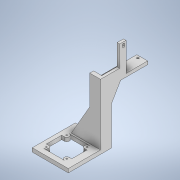
# Autodesk Inventor part: camera_mount_v1
Saved by Autodesk Inventor 2022 (Build 260153000, 153)
## iProperties
Created: 2022-06-05
Part Number: camera_mount_v1
Material: Generic
Document SubType Name: Modeling
Designer: kylem
Density: 1 g/cm^3
Appearance: Default
Author: kylem
Autodesk Inventor part; units mm, degrees
ref_plane "YZ Plane" through (0, 0, 0) normal (1, 0, 0) x (0, 1, 0)
ref_plane "XZ Plane" through (0, 0, 0) normal (0, 1, 0) x (-1, 0, 0)
ref_plane "XY Plane" through (0, 0, 0) normal (0, 0, 1) x (1, 0, 0)
sketch "Sketch1" plane through (0, 0, 0) normal (0, 1, 0) x (-1, 0, 0)
  line L0 (0, 0) -> (13, 0)
  line L1 (13, 0) -> (13, -44)
  line L2 (13, -44) -> (0, -44)
  line L3 (0, -44) -> (0, 0)
  line L4 (13, 0) -> (13, -6)
  line L5 (13, -6) -> (7.5, -6)
  line L6 (7.5, -6) -> (7.5, -40)
  circle A0 centre (7.5, -6) radius 1.6
  circle A1 centre (7.5, -40) radius 1.6
  dimension "d0" = 13
  dimension "d1" = 44
  dimension "d2" = 6
  dimension "d3" = 5.5
  dimension "d4" = 34
  dimension "d5" = 3.2
  dimension "d6" = 3.2
  constraints: 14 end point, 3 parallel, 2 centre point, 2 coincident, 2 perpendicular, 1 horizontal, 1 point on line
  measures "d0" distance of L1.end L2.end
  measures "d1" distance of L0.end L1.end
  measures "d2" distance of L0.end L4.end
  measures "d3" distance of L4.end L5.end
  measures "d4" distance of L5.end L6.end
  measures "d5" diameter of A0
  measures "d6" diameter of A1
extrude "Extrusion1" add sketch "Sketch1" along normal blind 5
sketch "Sketch2" plane through (0, 0, 0) normal (1, 0, 0) x (0, 0, -1)
  line L0 (0, 5) -> (44, 5) projected
  line L1 (0, 5) -> (44, 5)
  line L2 (44, 5) -> (44, 50)
  line L3 (44, 50) -> (0, 50)
  line L4 (0, 50) -> (0, 5)
  line L5 (0, 0) -> (44, 0)
  line L6 (44, 0) -> (44, 5)
  line L7 (44, 5) -> (0, 5)
  line L8 (0, 5) -> (0, 0)
  line L9 (0, 50) -> (10, 50)
  line L10 (10, 50) -> (10, 5)
  line L11 (10, 5) -> (0, 5)
  line L12 (0, 5) -> (0, 50)
  dimension "d9" = 44
  dimension "d10" = 45
  dimension "d11" = 10
  constraints: 24 end point, 6 parallel, 3 horizontal, 3 perpendicular, 1 point on line
  measures "d9" distance of L3.end L2.end
  measures "d10" distance of L2.end L1.end
  measures "d11" distance of L10.end L11.end
extrude "Extrusion2" add sketch "Sketch2" along normal blind 4 contours L4 L3 L10 L0 | L0 L6 L5 L8
sketch "Sketch3" plane through (4, 0, 0) normal (1, 0, 0) x (0, 0, -1)
  line L0 (44, 5) -> (10, 5) projected
  line L1 (10, 5) -> (10, 45)
  line L2 (10, 5) -> (10, 50) projected
  line L3 (0, 50) -> (0, 5) projected
  line L4 (0, 45) -> (4.4, 45)
  line L5 (6, 45) -> (6, 46.5)
  line L6 (6, 45) -> (6, 43.5)
  line L7 (4.4, 46.5) -> (4.4, 43.5)
  line L8 (7.6, 46.5) -> (7.6, 43.5)
  arc A0 (5.4432, 45) -> (6, 44.9) centre (6, 46.5) ccw
  arc A1 (6.5568, 45) -> (4.4, 46.5) centre (6, 46.5) ccw
  line L9 (10, 45) -> (6.5568, 45)
  line L10 (5.4432, 45) -> (0, 45)
  arc A2 (6, 45.1) -> (5.4432, 45) centre (6, 43.5) ccw
  arc A3 (4.4, 43.5) -> (7.6, 43.5) centre (6, 43.5) ccw
  point P0 (0, 0)
  dimension "d14" = 40
  dimension "d15" = 6
  dimension "d16" = 1.5
  dimension "d17" = 1.5
  constraints: 16 end point, 9 point on circle, 4 centre point, 4 tangent, 3 point on line, 2 coincident, 2 perpendicular, 2 vertical, 1 midpoint
  measures "d14" distance of L0.end L1.end
  measures "d15" distance of L4.start L5.start
  measures "d16" distance of L5.start L5.end
  measures "d17" distance of L5.start L6.end
extrude "Extrusion3" cut sketch "Sketch3" against normal blind 4 contours L6 A0 A2 L5 | A1 L9 L8 A3 L7 | L8 L9 A1
sketch "Sketch4" plane through (-13, 0, 0) normal (0, 0, 1) x (1, 0, 0)
  line L0 (0, 0) -> (17, 0) projected
  line L1 (17, 0) -> (17, 5) projected
  line L2 (0, 0) -> (17, 0)
  line L3 (17, 0) -> (17, 5)
  line L4 (17, 5) -> (0, 5)
  line L5 (0, 5) -> (0, 0)
  line L6 (13, 50) -> (13, 5) projected
  line L7 (17, 0) -> (13, 0)
  line L8 (13, 0) -> (13, 17)
  line L9 (13, 17) -> (17, 17)
  line L10 (17, 17) -> (17, 0)
  dimension "d22" = 17
  constraints: 16 end point, 4 parallel, 2 horizontal, 2 perpendicular, 1 point on line
  measures "d22" distance of L7.end L8.end
extrude "Extrusion4" add sketch "Sketch4" along normal blind 30
sketch "Sketch5" plane through (0, 0, 0) normal (0, -1, 0) x (1, 0, 0)
  line L0 (-13, -44) -> (-13, 30) projected
  line L1 (-13, 30) -> (4, 30)
  line L2 (4, 30) -> (4, 13)
  line L3 (4, 13) -> (-13, 13)
  line L4 (-13, 13) -> (-13, 30)
  point P0 (0, 0)
  dimension "d25" = 17
  dimension "d26" = 17
  constraints: 8 end point, 2 parallel, 1 horizontal, 1 perpendicular
  measures "d25" distance of L2.end L3.end
  measures "d26" distance of L1.end L2.end
extrude "Extrusion5" add sketch "Sketch5" along normal blind 85
sketch "Sketch7" plane through (0, -85, 0) normal (0, -1, 0) x (1, 0, 0)
  line L0 (4, 13) -> (-13, 13) projected
  line L1 (0, 30) -> (0, -10) projected
  line L2 (0, 13) -> (0, 30)
  line L3 (0, 30) -> (0, 52.6)
  circle A0 centre (-36, 52.6) radius 9
  line L4 (-36, 52.6) -> (-36, 36.6)
  line L5 (-36, 36.6) -> (-20, 36.6)
  line L6 (-36, 52.6) -> (-36, 68.6)
  line L7 (-36, 68.6) -> (-52, 68.6)
  line L8 (-52, 68.6) -> (-20, 68.6)
  line L9 (-20, 68.6) -> (-20, 36.6)
  line L10 (-20, 36.6) -> (-52, 36.6)
  line L11 (-52, 36.6) -> (-52, 68.6)
  circle A1 centre (-20, 68.6) radius 1.1
  circle A2 centre (-20, 36.6) radius 1.1
  circle A3 centre (-52, 36.6) radius 1.1
  circle A4 centre (-52, 68.6) radius 1.1
  circle A5 centre (-20, 68.6) radius 4
  circle A6 centre (-20, 36.6) radius 4
  line L12 (-52, 65.6) -> (-52, 70.6)
  line L13 (-52, 36.6) -> (-52, 42.6)
  circle A7 centre (-52, 68.6) radius 4
  circle A8 centre (-52, 36.6) radius 4
  point P0 (0, 0)
  point P1 (-20, 64.6)
  point P2 (-20, 40.6)
  dimension "d29" = 22.6
  dimension "d31" = 18
  dimension "d32" = 16
  dimension "d33" = 16
  dimension "d34" = 16
  dimension "d35" = 16
  dimension "d36" = 2.2
  dimension "d37" = 2.2
  dimension "d39" = 2.2
  dimension "d40" = 8
  dimension "d43" = 8
  dimension "d49" = 8
  dimension "d50" = 8
  constraints: 24 end point, 9 centre point, 8 coincident, 3 perpendicular, 3 point on line, 2 parallel, 2 vertical, 1 collinear, 1 horizontal
  measures "d29" distance of L1.start L3.end
  measures "d31" diameter of A0
  measures "d32" distance of L4.start L4.end
  measures "d33" distance of L4.end L5.end
  measures "d34" distance of L4.start L6.end
  measures "d35" distance of L6.end L7.end
  measures "d36" diameter of A1
  measures "d37" diameter of A2
  measures "d39" diameter of A4
  measures "d40" diameter of A5
  measures "d43" diameter of A6
  measures "d49" diameter of A7
  measures "d50" diameter of A8
sketch "Sketch14" plane through (0, -85, 0) normal (0, -1, 0) x (1, 0, 0)
  line L0 (4, 13) -> (4, 30) projected
  line L1 (4, 13) -> (4, 52.6)
  line L2 (4, 52.6) -> (-26.5, 52.6)
  line L3 (-26.5, 52.6) -> (-26.5, 36.6)
  line L4 (-26.5, 36.6) -> (-10.5, 36.6)
  line L5 (-26.5, 52.6) -> (-42.5, 52.6)
  line L6 (-42.5, 52.6) -> (-42.5, 68.6)
  line L7 (-42.5, 68.6) -> (-10.5, 68.6)
  line L8 (-10.5, 68.6) -> (-10.5, 36.6)
  line L9 (-10.5, 36.6) -> (-42.5, 36.6)
  line L10 (-42.5, 36.6) -> (-42.5, 68.6)
  circle A0 centre (-42.5, 68.6) radius 1.1
  circle A1 centre (-10.5, 68.6) radius 1.1
  circle A2 centre (-10.5, 36.6) radius 1.1
  circle A3 centre (-42.5, 36.6) radius 1.1
  circle A4 centre (-42.5, 68.6) radius 4
  circle A5 centre (-10.5, 68.6) radius 4
  circle A6 centre (-10.5, 36.6) radius 4
  circle A7 centre (-42.5, 36.6) radius 4
  point P0 (0, 0)
  dimension "d91" = 39.6
  dimension "d92" = 30.5
  dimension "d93" = 16
  dimension "d94" = 16
  dimension "d95" = 16
  dimension "d96" = 16
  dimension "d97" = 2.2
  dimension "d98" = 2.2
  dimension "d99" = 2.2
  dimension "d100" = 2.2
  dimension "d101" = 8
  dimension "d102" = 8
  dimension "d103" = 8
  dimension "d104" = 8
  constraints: 20 end point, 8 centre point, 8 coincident, 4 perpendicular, 2 horizontal, 2 parallel, 1 collinear, 1 vertical
  measures "d91" distance of L0.start L1.end
  measures "d92" distance of L1.end L2.end
  measures "d93" distance of L2.end L3.end
  measures "d94" distance of L3.end L4.end
  measures "d95" distance of L2.end L5.end
  measures "d96" distance of L5.end L6.end
  measures "d97" diameter of A0
  measures "d98" diameter of A1
  measures "d99" diameter of A2
  measures "d100" diameter of A3
  measures "d101" diameter of A4
  measures "d102" diameter of A5
  measures "d103" diameter of A6
  measures "d104" diameter of A7
extrude "Extrusion14" add sketch "Sketch14" against normal blind 6 contours A5 L7 A1 L8 | L8 A1 L7 A5 | A6 L4 A2 L8 | L8 A2 L4 A6 | A7 L10 A3 L9 | L9 A3 L10 A7 | A4 L7 A0 L6 | L6 A0 L7 A4
sketch "Sketch15" plane through (-10.5, -85, 68.6) normal (0, -1, 0) x (1, 0, 0)
  circle A0 centre (0, 0) radius 4 projected
  line L0 (0, 4) -> (10, 4)
  line L1 (10, 4) -> (10, -4)
  line L2 (10, -4) -> (0, -4)
  line L3 (0, -4) -> (0, 4)
  circle A1 centre (0, -32) radius 4 projected
  line L4 (0, -28) -> (10, -28)
  line L5 (10, -28) -> (10, -36)
  line L6 (10, -36) -> (0, -36)
  line L7 (0, -36) -> (0, -28)
  circle A2 centre (-32, -32) radius 4 projected
  line L8 (-32, -36) -> (-42, -36)
  line L9 (-42, -36) -> (-42, -28)
  line L10 (-42, -28) -> (-32, -28)
  line L11 (-32, -28) -> (-32, -36)
  circle A3 centre (-32, 0) radius 4 projected
  line L12 (-32, -4) -> (-42, -4)
  line L13 (-42, -4) -> (-42, 4)
  line L14 (-42, 4) -> (-32, 4)
  line L15 (-32, 4) -> (-32, -4)
  line L16 (-42, 4) -> (-36, 4)
  line L17 (-36, 4) -> (-36, -36)
  line L18 (-36, -36) -> (-42, -36)
  line L19 (-42, -36) -> (-42, 4)
  line L20 (10, 4) -> (4, 4)
  line L21 (4, 4) -> (4, -36)
  line L22 (4, -36) -> (10, -36)
  line L23 (10, -36) -> (10, 4)
  point P0 (10.5, -68.6)
  point P1 (-36, -4)
  point P2 (-32, 4)
  point P3 (-42, -4)
  point P4 (-36, -28)
  point P5 (0, -4)
  point P6 (4, -4)
  point P7 (4, -28)
  point P8 (10, -4)
  dimension "d107" = 10
  dimension "d108" = 8
  dimension "d109" = 10
  dimension "d110" = 8
  dimension "d111" = 10
  dimension "d112" = 8
  dimension "d113" = 10
  dimension "d114" = 8
  dimension "d115" = 6
  dimension "d116" = 6
  constraints: 48 end point, 12 parallel, 6 horizontal, 6 perpendicular, 5 point on line, 8 other
  measures "d107" distance of L1.end L2.end
  measures "d108" distance of L0.end L1.end
  measures "d109" distance of L5.end L6.end
  measures "d110" distance of L4.end L5.end
  measures "d111" distance of L9.end L10.end
  measures "d112" distance of L8.end L9.end
  measures "d113" distance of L13.end L14.end
  measures "d114" distance of L12.end L13.end
  measures "d115" distance of L17.end L18.end
  measures "d116" distance of L22.end L21.end
extrude "Extrusion15" add sketch "Sketch15" against normal blind 6 contours L21 L2 A0 | A0 L0 L21 | L21 L0 L1 L2 | L2 L23 L4 L21 | L21 A1 L4 | L4 L5 L6 L21 | L21 L6 A1 | A2 L17 L10 | L8 L17 A2 | L17 L8 L9 L10 | L10 L19 L12 L17 | L17 A3 L12 | L12 L13 L14 L17 | L17 L14 A3
sketch "Sketch16" plane through (0, -85, 0) normal (0, -1, 0) x (1, 0, 0)
  line L0 (-0.5, 72.6) -> (-0.5, 32.6) projected
  line L1 (-0.5, 72.6) -> (-52.5, 72.6)
  line L2 (-52.5, 72.6) -> (-52.5, 80.6)
  line L3 (-52.5, 80.6) -> (-0.5, 80.6)
  line L4 (-0.5, 80.6) -> (-0.5, 72.6)
  line L5 (-0.5, 32.6) -> (-10.5, 32.6) projected
  line L6 (-0.5, 32.6) -> (-52.5, 32.6)
  line L7 (-52.5, 32.6) -> (-52.5, 24.6)
  line L8 (-52.5, 24.6) -> (-0.5, 24.6)
  line L9 (-0.5, 24.6) -> (-0.5, 32.6)
  point P0 (0, 0)
  dimension "d119" = 8
  dimension "d120" = 8
  constraints: 16 end point, 4 parallel, 2 horizontal, 2 perpendicular
  measures "d119" distance of L1.end L2.end
  measures "d120" distance of L7.end L6.end
extrude "Extrusion16" add sketch "Sketch16" against normal blind 6
sketch "Sketch17" plane through (0, -79, 0) normal (0, 1, 0) x (1, 0, 0)
  line L0 (-0.5, -80.6) -> (-0.5, -30) projected
  line L1 (4, -30) -> (0, -30) projected
  line L2 (-0.5, -80.6) -> (4, -80.6)
  line L3 (4, -80.6) -> (4, -30)
  line L4 (4, -30) -> (-0.5, -30)
  line L5 (-0.5, -30) -> (-0.5, -80.6)
  line L6 (-52.5, -24.6) -> (-52.5, -80.6) projected
  line L7 (-52.5, -24.6) -> (-13, -24.6)
  line L8 (-13, -24.6) -> (-13, -13)
  line L9 (-13, -13) -> (-52.5, -13)
  line L10 (-52.5, -13) -> (-52.5, -24.6)
  point P0 (0, 0)
  constraints: 16 end point, 4 parallel, 2 horizontal, 2 perpendicular
extrude "Extrusion17" add sketch "Sketch17" against normal blind 6
chamfer "Chamfer4" distance 50 angle 30 1 edges at (-13, -79, 21.5) measured on face at (-13, -24.6667, 24.3333)
chamfer "Chamfer5" distance 25 angle 30 1 edges at (-4.5, 0, 13) measured on face at (-16.9558, -64.3333, 13)
sketch "Sketch19" plane through (-13, 0, 30) normal (0, 0, 1) x (1, 0, 0)
  line L0 (13, 17) -> (13, 5) projected
  line L1 (0, 0) -> (0, 5) projected
  line L2 (13, 17) -> (0, 17)
  line L3 (0, 17) -> (0, 5)
  line L4 (0, 5) -> (13, 5)
  line L5 (13, 5) -> (13, 17)
  point P0 (13, 0)
  constraints: 8 end point, 2 parallel, 1 horizontal, 1 perpendicular
extrude "Extrusion18" add sketch "Sketch19" against normal blind 6
body "Solid1"
